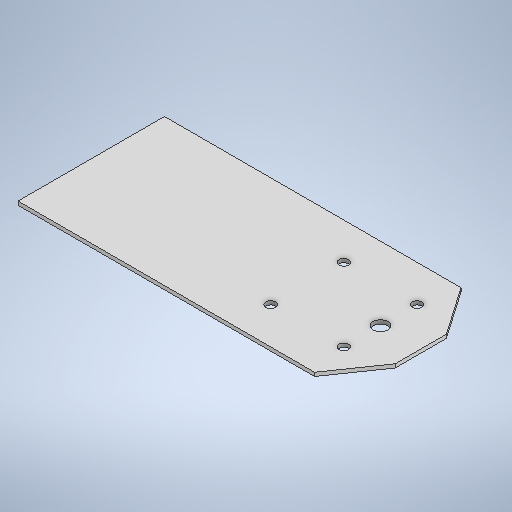
# Autodesk Inventor part: motorholder
Saved by Autodesk Inventor 2025.1 (Build 291241000, 241)
## iProperties
Created: 2025-11-11
Part Number: motorholder
Material: Generic
Document SubType Name: Modeling
Designer: mukund
Density: 1 g/cm^3
Appearance: Default
Author: mukund
Autodesk Inventor part; units mm, degrees
ref_plane "YZ Plane" through (0, 0, 0) normal (1, 0, 0) x (0, 1, 0)
ref_plane "XZ Plane" through (0, 0, 0) normal (0, 1, 0) x (-1, 0, 0)
ref_plane "XY Plane" through (0, 0, 0) normal (0, 0, 1) x (1, 0, 0)
sketch "Sketch1" plane through (0, 0, 0) normal (0, 1, 0) x (-1, 0, 0)
  line L0 (-90, -40) -> (90, -40)
  line L1 (90, -40) -> (90, 40)
  line L2 (90, 40) -> (-90, 40)
  line L3 (-90, 40) -> (-90, -40)
  line L4 (-90, -40) -> (90, 40) construction
  line L5 (90, -40) -> (-90, 40) construction
  line L6 (90, 40) -> (90, 20)
  line L7 (90, 20) -> (-28, 20)
  line L8 (-28, 20) -> (-28, -20)
  line L9 (-28, -20) -> (-68, -20)
  line L10 (-68, -20) -> (-68, 20)
  line L11 (-68, 20) -> (-28, 20)
  line L12 (90, -40) -> (-72, -40)
  line L13 (90, 40) -> (-72, 40)
  line L14 (-90, 0) -> (-90, 14)
  line L15 (-90, 14) -> (-72, 40)
  line L16 (-90, 0) -> (-90, -14)
  line L17 (-90, -14) -> (-72, -40)
  circle A0 centre (-68, 20) radius 2.6
  circle A1 centre (-68, -20) radius 2.6
  circle A2 centre (-28, -20) radius 2.6
  circle A3 centre (-28, 20) radius 2.6
  circle A4 centre (-68, 0) radius 4
  point P0 (0, 0)
  dimension "d0" = 180
  dimension "d1" = 80
  dimension "d2" = 20
  dimension "d3" = 118
  dimension "d4" = 40
  dimension "d5" = 40
  dimension "d6" = 162
  dimension "d7" = 162
  dimension "d8" = 14
  dimension "d9" = 14
  dimension "d10" = 5.2
  dimension "d11" = 5.2
  dimension "d12" = 5.2
  dimension "d13" = 5.2
  dimension "d14" = 8
  constraints: 36 end point, 6 point on line, 5 centre point, 5 perpendicular, 4 coincident, 4 midpoint, 2 parallel, 1 collinear, 1 horizontal
  measures "d0" distance of L2.end L1.end
  measures "d1" distance of L1.end L0.end
  measures "d2" distance of L1.end L6.end
  measures "d3" distance of L6.end L7.end
  measures "d4" distance of L7.end L8.end
  measures "d5" distance of L8.end L9.end
  measures "d6" distance of L0.end L12.end
  measures "d7" distance of L1.end L13.end
  measures "d8" distance of L14.start L14.end
  measures "d9" distance of L14.start L16.end
  measures "d10" diameter of A0
  measures "d11" diameter of A1
  measures "d12" diameter of A2
  measures "d13" diameter of A3
  measures "d14" diameter of A4
extrude "Extrusion1" add sketch "Sketch1" along normal blind 2 contours L17 L3 L15 L2 L1 L0 | A3 L8 A2 L9 A1 L10 A4 A0 L11
body "Solid1"
